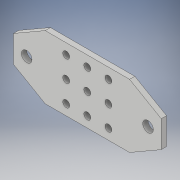
# Autodesk Inventor part: piece
Saved by Autodesk Inventor 2018 (Build 220112000, 112)
## iProperties
Created: 2018-08-29
Part Number: piece
Material: Generic
Document SubType Name: Modeling
Designer: baoan
Density: 1 g/cm^3
Appearance: Default
Author: baoan
Autodesk Inventor part; units mm, degrees
ref_plane "YZ Plane" through (0, 0, 0) normal (1, 0, 0) x (0, 1, 0)
ref_plane "XZ Plane" through (0, 0, 0) normal (0, 1, 0) x (-1, 0, 0)
ref_plane "XY Plane" through (0, 0, 0) normal (0, 0, 1) x (1, 0, 0)
sketch "Sketch1" plane through (0, 0, 0) normal (0, 0, 1) x (1, 0, 0)
  line L0 (44.45, -19.05) -> (25.4, -19.05) construction
  line L1 (-44.45, -19.05) -> (-44.45, -8.0515) construction
  line L2 (-44.45, 19.05) -> (-25.4, 19.05) construction
  line L3 (44.45, 19.05) -> (44.45, 8.0515) construction
  line L4 (44.45, -19.05) -> (-44.45, 19.05) construction
  line L5 (-44.45, -19.05) -> (44.45, 19.05) construction
  line L6 (-44.45, 8.0515) -> (-25.4, 19.05)
  line L7 (0, 16.7111) -> (0, 5.8205) construction
  line L8 (44.45, 8.0515) -> (25.4, 19.05)
  line L9 (-44.45, 0) -> (-27.1015, 0) construction
  line L10 (-44.45, -8.0515) -> (-25.4, -19.05)
  line L11 (44.45, -8.0515) -> (25.4, -19.05)
  line L12 (-25.4, 19.05) -> (25.4, 19.05)
  line L13 (-44.45, 8.0515) -> (-44.45, 19.05) construction
  line L14 (-25.4, -19.05) -> (-44.45, -19.05) construction
  line L15 (-44.45, -8.0515) -> (-44.45, 8.0515)
  line L16 (25.4, -19.05) -> (-25.4, -19.05)
  line L17 (44.45, -8.0515) -> (44.45, -19.05) construction
  line L18 (44.45, 8.0515) -> (44.45, -8.0515)
  line L19 (25.4, 19.05) -> (44.45, 19.05) construction
  circle A0 centre (-12.7, 12.7) radius 2.0701
  circle A1 centre (12.7, -12.7) radius 2.0701
  circle A2 centre (0, -12.7) radius 2.0701
  circle A3 centre (-12.7, -12.7) radius 2.0701
  circle A4 centre (12.7, 0) radius 2.0701
  circle A5 centre (0, 0) radius 2.0701
  circle A6 centre (-12.7, 0) radius 2.0701
  circle A7 centre (12.7, 12.7) radius 2.0701
  circle A8 centre (0, 12.7) radius 2.0701
  circle A9 centre (-36.5125, 0) radius 3.2004
  circle A10 centre (36.5125, 0) radius 3.2004
  line L20 (-36.5125, 0) -> (36.5125, 0)
  point P0 (0, 0)
  point P1 (0, 12.7)
  point P2 (12.7, 12.7)
  point P3 (12.7, 0)
  point P4 (0, 0)
  point P5 (-12.7, 0)
  point P6 (-12.7, -12.7)
  point P7 (0, -12.7)
  point P8 (12.7, -12.7)
  point P9 (0, 0)
  point P10 (0, 0)
  dimension "d0" = 88.9
  dimension "d1" = 38.1
  dimension "d2" = 150
  dimension "d3" = 19.05
  dimension "d6" = 6.35
  dimension "d7" = 12.7
  dimension "d8" = 12.7
  dimension "d9" = 12.7
  dimension "d10" = 12.7
  dimension "d11" = 4.1402
  dimension "d12" = 4.1402
  dimension "d13" = 4.1402
  dimension "d14" = 4.1402
  dimension "d15" = 4.1402
  dimension "d16" = 4.1402
  dimension "d17" = 4.1402
  dimension "d18" = 4.1402
  dimension "d19" = 4.1402
  dimension "d20" = 73.025
  dimension "d22" = 6.4008
  dimension "d23" = 6.4008
  constraints: 42 end point, 18 parallel, 12 coincident, 11 centre point, 9 perpendicular, 8 horizontal alignment, 7 vertical alignment, 6 symmetric about line, 4 horizontal, 4 midpoint, 1 collinear, 1 vertical
  measures "d0" distance of L2.start L3.start
  measures "d1" distance of L1.start L2.start
  measures "d2" angle of L2 L6
  measures "d3" distance from line of L1 L2.end
  measures "d6" distance from line of L12 point (0, 12.7)
  measures "d7" distance of point (12.7, 12.7) point (0, 12.7)
  measures "d8" distance of point (-12.7, 12.7) point (0, 12.7)
  measures "d9" distance of point (0, 12.7) point (0, 0)
  measures "d10" distance of point (0, 0) point (0, -12.7)
  measures "d11" diameter of A0
  measures "d12" diameter of A1
  measures "d13" diameter of A2
  measures "d14" diameter of A3
  measures "d15" diameter of A4
  measures "d16" diameter of A5
  measures "d17" diameter of A6
  measures "d18" diameter of A7
  measures "d19" diameter of A8
  measures "d20" distance of point (36.513, 0) point (-36.513, 0)
  measures "d22" diameter of A9
  measures "d23" diameter of A10
extrude "Extrusion2" add sketch "Sketch1" along normal mid plane 3.175
body "Solid2"
